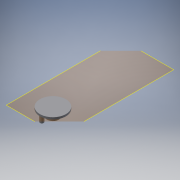
# Autodesk Inventor part: Cup_Dispenser_Transmission
Saved by Autodesk Inventor 2016 (Build 200138000, 138)
## iProperties
Created: 2015-07-04
Part Number: Cup_Dispenser_Transmission
Material: Generic
Document SubType Name: Modeling
Designer: marku
Density: 1 g/cm^3
Appearance: Default
Author: marku
Autodesk Inventor part; units mm, degrees
ref_plane "YZ Plane" through (0, 0, 0) normal (1, 0, 0) x (0, 1, 0)
ref_plane "XZ Plane" through (0, 0, 0) normal (0, 1, 0) x (-1, 0, 0)
ref_plane "Work Plane1" through (0, 0, 0) normal (0, 0, 1) x (1, 0, 0)
sketch "Sketch1" plane through (0, 0, 0) normal (0, 0, 1) x (1, 0, 0)
  circle A0 centre (0, -82) radius 2.5 projected
  circle A1 centre (0, -82) radius 11.5 construction
  circle A2 centre (0, -82) radius 9.5
  circle A3 centre (0, -99.5) radius 3
  point P0 (0, 0)
  dimension "d0" = 2
  dimension "d5" = 6
  constraints: 2 centre point, 1 coincident
  measures "d0" radial gap between concentric circles of A1 A2
  measures "d5" diameter of A3
extrude "Extrusion1" add sketch "Sketch1" against normal blind 10
sketch "Sketch2" plane through (0, -82, 0) normal (0, 0, 1) x (1, 0, 0)
  circle A0 centre (0, 0) radius 17.5 construction
  circle A1 centre (0, 0) radius 20.5
  point P0 (0, 82)
  point P1 (0, -17.5)
  dimension "d6" = 3
  constraints: 1 centre point, 1 vertical alignment, 2 other
extrude "Extrusion2" add sketch "Sketch2" along normal blind 3
chamfer "Chamfer1" distance 1 angle 45 1 edges at (-3, -99.5, -10)
sketch "Sketch3" plane through (0, -82, 3) normal (0, 0, 1) x (1, 0, 0)
  circle A0 centre (0, 0) radius 20.5 projected
  circle A1 centre (0, 0) radius 2.5 projected
  point P0 (0, 82)
ref_plane "Work Plane2" through (-3.7976, -85.7976, 4.5) normal (0, 0, 1) x (1, 0, 0)
extrude "Extrusion3" add sketch "Sketch3" along normal up to surface (1.5 mm away)
sketch "Sketch4" plane through (0, -82, 4.5) normal (0, 0, 1) x (1, 0, 0)
  circle A0 centre (0, 0) radius 20.5 projected
  point P0 (0, 82)
extrude "Extrusion4" add sketch "Sketch4" along normal blind 3
body "Solid1"
